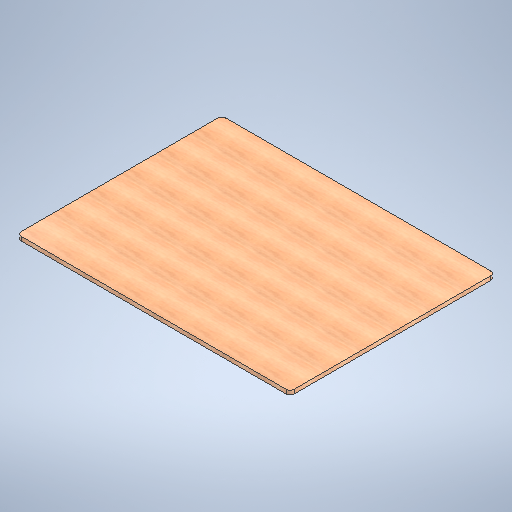
# Autodesk Inventor part: maquete_001_001
Saved by Autodesk Inventor 2026 (Build 300175000, 175)
## iProperties
Created: 2025-05-22
Part Number: maquete_001_001
Material: Wood (Birch)
Document SubType Name: Modeling
Designer: carlo
Density: 0.55 g/cm^3
Appearance: Birch - Natural Polished
Author: carlo
Autodesk Inventor part; units mm, degrees
sketch "Sketch2" plane through (0, 0, 0) normal (0, 1, 0) x (-1, 0, 0)
  line L0 (1000, -750) -> (-1000, -750)
  line L1 (-1000, -750) -> (-1000, 750)
  line L2 (-1000, 750) -> (1000, 750)
  line L3 (1000, 750) -> (1000, -750)
  line L4 (1000, -750) -> (-1000, 750) construction
  line L5 (-1000, -750) -> (1000, 750) construction
  point P0 (0, 0)
  dimension "d0" = 2000
  dimension "d1" = 1500
  constraints: 12 end point, 2 midpoint, 2 parallel, 1 horizontal, 1 perpendicular
  measures "d0" distance of L1.end L2.end
  measures "d1" distance of L0.end L1.end
extrude "Extrusion1" add sketch "Sketch2" against normal blind 30
fillet "Fillet1" radius 30 4 edges at (1000, -15, -750) (1000, -15, 750) (-1000, -15, 750) (-1000, -15, -750)
body "Solid1"
